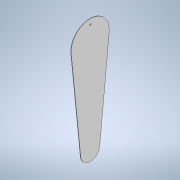
# Autodesk Inventor part: main_plate
Saved by Autodesk Inventor 2022.5 (Build 265521000, 521)
## iProperties
Created: 2024-06-27
Part Number: main_plate
Material: 一般
Document SubType Name: Modeling
Designer: gakut
Density: 1 g/cm^3
Appearance: 既定
Author: gakut
Autodesk Inventor part; units mm, degrees
ref_plane "YZ Plane" through (0, 0, 0) normal (1, 0, 0) x (0, 1, 0)
ref_plane "XZ Plane" through (0, 0, 0) normal (0, 1, 0) x (-1, 0, 0)
ref_plane "XY Plane" through (0, 0, 0) normal (0, 0, 1) x (1, 0, 0)
sketch "スケッチ1" plane through (0, 0, 0) normal (1, 0, 0) x (0, 1, 0)
  circle A0 centre (0, 0) radius 40
  dimension "d0" = 80
  constraints: 1 centre point, 1 coincident
  measures "d0" diameter of A0
extrude "押し出し1" add sketch "スケッチ1" along normal blind 1
sketch "スケッチ2" plane through (1, 0, 0) normal (1, 0, 0) x (0, 0, -1)
  point P0 (0, 0)
  point P1 (0, 29)
  dimension "d3" = 29
  constraints: 1 vertical alignment
  measures "d3" distance of point (0, 0) point (0, 29)
hole "穴1" at (1, 29, 0) direction (-1, 0, 0) diameter 4 end through all
sketch "スケッチ4" plane through (1, 0, 0) normal (1, 0, 0) x (0, 0, -1)
  circle A0 centre (0, -200) radius 20
  circle A1 centre (0, 0) radius 40 projected
  line L0 (-39.7995, -4) -> (-19.8997, -202)
  line L1 (39.7995, -4) -> (19.8997, -202)
  circle A2 centre (0, 0) radius 40 projected
  dimension "d13" = 40
  dimension "d14" = 200
  constraints: 4 end point, 4 point on circle, 4 tangent, 1 centre point, 1 vertical alignment
  measures "d13" diameter of A0
  measures "d14" distance of A0.centre point (0, 0)
extrude "押し出し2" add sketch "スケッチ4" against normal blind 1 contours A0 | A0 L0 A1 L1
sketch "スケッチ5" plane through (0, 0, 0) normal (-1, 0, 0) x (0, 0, 1)
  line L0 (-14.3506, 34.6455) -> (14.3506, 34.6455)
  line L1 (14.3506, 34.6455) -> (34.6455, 14.3506)
  line L2 (34.6455, 14.3506) -> (34.6455, -14.3506)
  line L3 (34.6455, -14.3506) -> (14.3506, -34.6455)
  line L4 (14.3506, -34.6455) -> (-14.3506, -34.6455)
  line L5 (-14.3506, -34.6455) -> (-34.6455, -14.3506)
  line L6 (-34.6455, -14.3506) -> (-34.6455, 14.3506)
  line L7 (-34.6455, 14.3506) -> (-14.3506, 34.6455)
  circle A0 centre (0, 29) radius 2 projected
  line L8 (0, 0) -> (0, 29)
  dimension "d17" = 37.5
  constraints: 18 end point, 1 coincident, 1 perpendicular, 1 vertical, 17 other
  measures "d17" distance of L0.end L8.start
hole "穴2" at (0, 34.6455, -14.3506) at (0, 14.3506, -34.6455) at (0, -14.3506, -34.6455) at (0, -34.6455, -14.3506) at (0, -34.6455, 14.3506) at (0, -14.3506, 34.6455) at (0, 14.3506, 34.6455) at (0, 34.6455, 14.3506) direction (1, 0, 0) diameter 3 end through all
